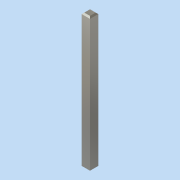
# Autodesk Inventor part: Pin
Saved by Autodesk Inventor 2017 (Build 210142000, 142)
## iProperties
Created: 2017-01-25
Part Number: Pin
Material: Silver
Document SubType Name: Modeling
Designer: techn
Density: 10.49 g/cm^3
Appearance: Silver
Author: techn
Autodesk Inventor part; units mm, degrees
ref_plane "YZ Plane" through (0, 0, 0) normal (1, 0, 0) x (0, 1, 0)
ref_plane "XZ Plane" through (0, 0, 0) normal (0, 1, 0) x (-1, 0, 0)
ref_plane "XY Plane" through (0, 0, 0) normal (0, 0, 1) x (1, 0, 0)
sketch "Sketch3" plane through (0, 0, 0) normal (0, 0, 1) x (1, 0, 0)
  line L0 (0, 0) -> (0.65, 0)
  line L1 (0.65, 0) -> (0.65, 6)
  line L2 (0.65, 6) -> (0, 6)
  line L3 (0, 6) -> (0, 0)
  line L4 (0.325, 0) -> (2.865, 0)
  line L5 (0, 0) -> (0.65, 0)
  line L6 (0.65, 0) -> (0.65, -4.5)
  line L7 (0.65, -4.5) -> (0, -4.5)
  line L8 (0, -4.5) -> (0, 0)
  dimension "d0" = 0.65
  dimension "d1" = 6
  dimension "d3" = 4.5
  constraints: 18 end point, 4 parallel, 3 horizontal, 2 perpendicular, 1 midpoint, 1 point on line
  measures "d0" distance of L2.end L1.end
  measures "d1" distance of L1.end L0.end
  measures "d3" distance of L5.end L6.end
extrude "Extrusion1" add sketch "Sketch3" along normal blind 0.65
chamfer "Chamfer1" distance 0.1 angle 45 8 edges at (0.65, 6, 0.325) (0.325, 6, 0.65) (0, 6, 0.325) (0.325, 6, 0) (0.65, -4.5, 0.325) (0.325, -4.5, 0.65) (0, -4.5, 0.325) (0.325, -4.5, 0)
body "Solid1"
